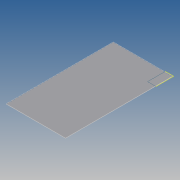
# Autodesk Inventor part: Bandeja recolectora
Saved by Autodesk Inventor 2016 (Build 200138000, 138)
## iProperties
Created: 2016-05-26
Part Number: Bandeja recolectora
Material: Generic
Document SubType Name: Modeling
Designer: Familia
Density: 1 g/cm^3
Appearance: Default
Mass: 10.53 g
Surface Area: 424.23 cm^2
Volume: 10.53 cm^3
Author: Familia
Autodesk Inventor part; units mm, degrees
ref_plane "YZ Plane" through (0, 0, 0) normal (1, 0, 0) x (0, 1, 0)
ref_plane "XZ Plane" through (0, 0, 0) normal (0, 1, 0) x (-1, 0, 0)
ref_plane "Work Plane1" through (0, 0, 0) normal (0, 0, 1) x (1, 0, 0)
sketch "Sketch1" plane through (0, 0, 0) normal (0, 0, 1) x (1, 0, 0)
  line L0 (6.4345, -180.25) -> (6.4345, -145.25) projected
  line L1 (6.4345, 14.75) -> (6.4345, -14.75) projected
  line L2 (-101.5655, -150.75) -> (-101.5655, -180.25) projected
  line L3 (-101.5655, 14.75) -> (-101.5655, -20.25) projected
  line L4 (6.4345, -180.25) -> (-101.5655, -180.25)
  line L5 (-101.5655, 14.75) -> (6.4345, 14.75)
  line L6 (-101.5655, -150.75) -> (-101.5655, -20.25)
  line L7 (6.4345, -145.25) -> (6.4345, -14.75)
  point P0 (0, 0)
  constraints: 8 end point, 1 collinear, 1 horizontal, 1 vertical
extrude "Extrusion1" add sketch "Sketch1" along normal blind 0.5
body "Solid1"
